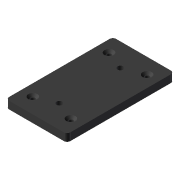
# Autodesk Inventor part: Encoder base
Saved by Autodesk Inventor 2020 (Build 240168000, 168)
## iProperties
Created: 2021-06-01
Part Number: Encoder base
Material: Generic
Document SubType Name: Modeling
Designer: ferrerx
Density: 1 g/cm^3
Appearance: Default
Author: ferrerx
Autodesk Inventor part; units mm, degrees
ref_plane "YZ Plane" through (0, 0, 0) normal (1, 0, 0) x (0, 1, 0)
ref_plane "XZ Plane" through (0, 0, 0) normal (0, 1, 0) x (-1, 0, 0)
ref_plane "XY Plane" through (0, 0, 0) normal (0, 0, 1) x (1, 0, 0)
sketch "Sketch1" plane through (0, 0, 0) normal (0, 1, 0) x (-1, 0, 0)
  line L0 (-20, 35) -> (20, 35)
  line L1 (20, 35) -> (20, -35)
  line L2 (20, -35) -> (-20, -35)
  line L3 (-20, -35) -> (-20, 35)
  line L4 (-20, 35) -> (20, -35) construction
  line L5 (20, 35) -> (-20, -35) construction
  circle A0 centre (0, 20) radius 2
  circle A1 centre (0, -20) radius 2
  line L6 (-12.5, 25) -> (12.5, 25) construction
  line L7 (12.5, 25) -> (12.5, -25) construction
  line L8 (12.5, -25) -> (-12.5, -25) construction
  line L9 (-12.5, -25) -> (-12.5, 25) construction
  line L10 (-12.5, 25) -> (12.5, -25) construction
  line L11 (12.5, 25) -> (-12.5, -25) construction
  circle A2 centre (12.5, -25) radius 5 construction
  circle A3 centre (12.5, -25) radius 1.5
  circle A4 centre (12.5, 25) radius 1.5
  circle A5 centre (-12.5, 25) radius 1.5
  circle A6 centre (-12.5, -25) radius 1.5
  point P0 (0, 0)
  dimension "d0" = 4
  dimension "d1" = 4
  dimension "d2" = 40
  dimension "d3" = 20
  dimension "d4" = 70
  dimension "d5" = 40
  dimension "d6" = 25
  dimension "d7" = 50
  dimension "d8" = 10
  dimension "d9" = 3
  dimension "d10" = 3
  dimension "d11" = 3
  dimension "d12" = 3
  constraints: 24 end point, 7 centre point, 5 coincident, 4 midpoint, 4 parallel, 2 horizontal, 2 perpendicular
  measures "d0" diameter of A0
  measures "d1" diameter of A1
  measures "d2" distance of A1.centre A0.centre
  measures "d3" distance of point (0, 0) A0.centre
  measures "d4" distance of L2.end L0.start
  measures "d5" distance of L1.end L2.end
  measures "d6" distance of L7.end L8.end
  measures "d7" distance of L8.end L6.start
  measures "d8" diameter of A2
  measures "d9" diameter of A4
  measures "d10" diameter of A5
  measures "d11" diameter of A6
  measures "d12" diameter of A3
extrude "Extrusion1" add sketch "Sketch1" along normal blind 5
fillet "Fillet1" radius 2 4 edges at (20, 2.5, 35) (20, 2.5, -35) (-20, 2.5, -35) (-20, 2.5, 35)
chamfer "Chamfer1" distance 1.5 angle 45 4 edges at (-11, 5, 25) (14, 5, 25) (-11, 5, -25) (14, 5, -25)
body "Solid1"
